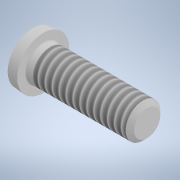
# Autodesk Inventor part: M2x6_b
Saved by Autodesk Inventor 2021 (Build 250183000, 183)
## iProperties
Created: 2025-06-07
Part Number: M2x6_b
Material: Generic
Catalog Web Link: www.cadenas.de
Description: H6-Rail Mount Screw
Vendor: MISUMI
Document SubType Name: Modeling
Designer: psAdmin
Manufacturer: MISUMI
Mass: 0.0217245 g
Surface Area: 0.591865 cm^2
Volume: 0.0217245 cm^3
Density: 1 g/cm^3
Appearance: PSOLRGB-175-175-175
Category: PARTsolutions
Company: MISUMI
Title: M2x6
Author: Cadenas PARTsolutions
Comments: Rail Mount Screw
PSOL_IDENT_0: {$CADENAS_DATA/23d-libs/misumi/metric/06_linear_guides/screw1.prj},146 {VTYP=3D},{NB=M2x6_b},{LINA=M
PSOL_IDENT_1: 2x6},{NN=H6},{DATE=29.11.2024 04:06:43},{GEOMDATE=15.10.2013 05:01:00},{VERSION=},{LINEID=10},{WBVAR=
PSOL_IDENT_2: },{WBNUMERIC=}  {NB=M2x6_b},{LINA=M2x6},{KT=DUMMY},{PN=M2x6},{DD=2.0},{PITCH=0.40},{D=3.0},{DTOL=+0.
PSOL_IDENT_3: 05/-0.1},{H=0.6},{HTOL=+/-0.05},{R=0.2},{M=2.00},{Q=1.21},{RR=0.05},{L=6},{W=0.6}
NB: M2x6_b
NN: H6
NT: Rail Mount Screw
NBSYN: $PN._b
LINA: M2x6
CATALOG: Misumi
PN: M2x6
DD: 2
PITCH: 0.4
D: 3
DTOL: +0.05/-0.1
H: 0.6
HTOL: +/-0.05
M: 2
Q: 1.21
L: 6
SUPPLIER: MISUMI
ARTICLENO: M2x6_b
BOMINFO: M2x6
CREATOR: CADENAS GmbH
Autodesk Inventor part; units mm, degrees
sketch "Sketch_1" plane through (0, 0, 0) normal (0, 0, 1) x (1, 0, 0)
  line L0 (6, 0) -> (-0.6, 0)
  line L1 (-0.6, 0) -> (-0.6, 1.5)
  line L2 (-0.6, 1.5) -> (0, 1.5)
  line L3 (0, 1.5) -> (0, 1.05)
  arc A0 (0, 1.05) -> (0.05, 1) centre (0.05, 1.05) ccw
  line L4 (0.05, 1) -> (5.7545, 1)
  line L5 (5.7545, 1) -> (6, 0.7545)
  line L6 (6, 0.7545) -> (6, 0)
  line L7 (6, 0) -> (-0.6, 0)
  constraints: 16 end point, 2 point on circle, 1 centre point
revolve "Revolution1" add sketch "Sketch_1" angle 360 about axis through (6, 0, 0) along (1, 0, 0)
thread "Thread1" size "M2x0.4" class "6g" standard "ISO Metric profile" length 5.3545
sketch "Sketch_3" plane through (0, 0, 0) normal (0, 0, 1) x (1, 0, 0)
  line L0 (0.61, 0) -> (-0.6, 0)
  line L1 (-0.6, 0) -> (-0.6, 1)
  line L2 (-0.6, 1) -> (0.61, 0)
  line L3 (0.61, 0) -> (-0.6, 0)
  constraints: 8 end point
revolve "Revolution2" cut sketch "Sketch_3" angle 360 about axis through (0.61, 0, 0) along (1, 0, 0)
sketch "Sketch_5" plane through (-0.6, 0, 0) normal (1, 0, 0) x (0, 0, -1)
  circle A0 centre (0, 0) radius 1.1
  arc A1 (-0.9539, 0.3) -> (-0.9539, -0.3) centre (0, 0) ccw
  line L0 (-0.9539, -0.3) -> (-0.3, -0.3)
  line L1 (-0.3, -0.3) -> (-0.3, -0.9539)
  arc A2 (-0.3, -0.9539) -> (0.3, -0.9539) centre (0, 0) ccw
  line L2 (0.3, -0.9539) -> (0.3, -0.3)
  line L3 (0.3, -0.3) -> (0.9539, -0.3)
  arc A3 (0.9539, -0.3) -> (0.9539, 0.3) centre (0, 0) ccw
  line L4 (0.9539, 0.3) -> (0.3, 0.3)
  line L5 (0.3, 0.3) -> (0.3, 0.9539)
  arc A4 (0.3, 0.9539) -> (-0.3, 0.9539) centre (0, 0) ccw
  line L6 (-0.3, 0.9539) -> (-0.3, 0.3)
  line L7 (-0.3, 0.3) -> (-0.9539, 0.3)
  constraints: 16 end point, 8 point on circle, 5 centre point
extrude "Extrusion1" add sketch "Sketch_5" along normal blind 0.3
sketch "Sketch_6" plane through (0, 0, 0) normal (0, 0, 1) x (1, 0, 0)
  line L0 (50, 0) -> (-50, 0)
  line L1 (-0.6, 1.5) -> (-0.6, 1.4475)
  line L2 (-0.6, 1.4475) -> (0, 1.5)
  line L3 (0, 1.5) -> (-0.6, 1.5)
  constraints: 8 end point
revolve "Revolution3" cut sketch "Sketch_6" angle 360 about axis through (50, 0, 0) along (1, 0, 0)
ref_plane "screw_to_rail_XY" through (0, 0, 0) normal (-1, 0, 0) x (0, 0, -1)
ref_plane "screw_to_rail_YZ" through (0, 0, 0) normal (0, 0, -1) x (0, -1, 0)
ref_plane "screw_to_rail_ZX" through (0, 0, 0) normal (0, -1, 0) x (-1, 0, 0)
body "Solid1"
